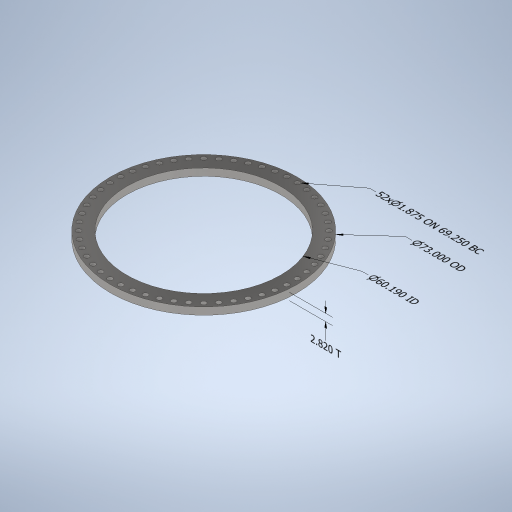
# Autodesk Inventor part: AWWA C207-18 Class B Ring and Blind Flange
Saved by Autodesk Inventor 2023 (Build 270158000, 158)
## iProperties
RuleStatus: InUse
Created: 2023-06-05
Part Number: AWWA C207-18 Class B Ring and Blind Flange
Material: Generic
Document SubType Name: Modeling
Designer: Admin
Density: 1 g/cm^3
Appearance: Steel - Polished
Author: Admin
Autodesk Inventor part; units mm, degrees
ref_plane "YZ Plane" through (0, 0, 0) normal (1, 0, 0) x (0, 1, 0)
ref_plane "XZ Plane" through (0, 0, 0) normal (0, 1, 0) x (-1, 0, 0)
ref_plane "XY Plane" through (0, 0, 0) normal (0, 0, 1) x (1, 0, 0)
sketch "Flange Sketch" plane through (0, 0, 0) normal (0, 1, 0) x (-1, 0, 0)
  circle A0 centre (0, 0) radius 927.1
  circle A1 centre (0, 0) radius 764.413
  circle A2 centre (0, 0) radius 879.475 construction
  line L0 (0, 0) -> (-53.1014, -877.8704) construction
  line L1 (0, 0) -> (0, -879.475) construction
  dimension "outerDiam" = 1854.2
  dimension "innerDiam" = 1528.826
  dimension "boltCircle" = 1758.95
  dimension "boltOffsetAngle" = 3.462
  constraints: 4 end point, 3 centre point, 3 coincident, 2 point on circle, 1 vertical
  measures "outerDiam" diameter of A0
  measures "innerDiam" diameter of A1
  measures "boltCircle" diameter of A2
  measures "boltOffsetAngle" angle of L0 L1
extrude "Flange Extrusion" add sketch "Flange Sketch" along normal blind 71.628
hole "Bolt Hole" at (53.1014, 0, -877.8704) direction (0, 1, 0) diameter 47.625 depth 71.628
pattern_circular "Bolt Hole Pattern" count 52 over 360 about axis through (0, -10, 0) along (0, 1, 0) of "Bolt Hole"
equation "\"nominalSize\" = 1524"
body "Solid1"
